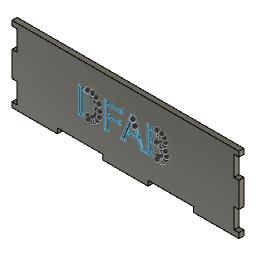
Component1 (Autodesk Fusion 360 design; units mm, degrees)
Autodesk Fusion 360 part; units mm, degrees
sketch "Sketch1" plane through (0, 0, 0) normal (0, 1, 0) x (1, 0, 0)
  line L0 (0, 0) -> (90, 0)
  line L1 (90, 0) -> (90, -30)
  line L2 (90, -30) -> (0, -30)
  line L3 (0, -30) -> (0, 0)
  line L4 (0, 0) -> (18, 0)
  line L5 (18, 0) -> (18, -2)
  line L6 (0, -2) -> (0, 0)
  line L7 (18, 0) -> (36, 0)
  line L8 (36, 0) -> (36, -2)
  line L9 (36, -2) -> (18, -2)
  line L10 (18, -2) -> (18, 0)
  line L11 (36, 0) -> (54, 0)
  line L12 (54, 0) -> (54, -2)
  line L13 (54, -2) -> (36, -2)
  line L14 (36, -2) -> (36, 0)
  line L15 (54, 0) -> (72, 0)
  line L16 (72, 0) -> (72, -2)
  line L17 (72, -2) -> (54, -2)
  line L18 (54, -2) -> (54, 0)
  line L19 (72, 0) -> (90, 0)
  line L20 (90, 0) -> (90, -2)
  line L21 (90, -2) -> (72, -2)
  line L22 (72, -2) -> (72, 0)
  line L23 (0, -30) -> (3, -30)
  line L24 (0, -30) -> (2, -30)
  line L25 (2, -30) -> (2, -20)
  line L26 (2, -20) -> (0, -20)
  line L27 (0, -20) -> (0, -30)
  line L28 (0, -20) -> (2, -20)
  line L29 (2, -20) -> (2, -10)
  line L30 (2, -10) -> (0, -10)
  line L31 (0, -10) -> (0, -20)
  line L32 (2, 0) -> (0, 0)
  line L33 (0, 0) -> (0, -10)
  line L34 (18, -2) -> (0, -2)
  line L35 (2, -10) -> (2, 0)
  line L36 (0, -10) -> (2, -10)
  line L37 (90, -30) -> (88, -30)
  line L38 (88, -30) -> (88, -20)
  line L39 (88, -20) -> (90, -20)
  line L40 (90, -20) -> (90, -30)
  line L41 (88, -20) -> (90, -20)
  line L42 (90, -20) -> (90, -10)
  line L43 (90, -10) -> (88, -10)
  line L44 (88, -10) -> (88, -20)
  line L45 (88, -10) -> (90, -10)
  line L46 (90, -10) -> (90, 0)
  line L47 (90, 0) -> (88, 0)
  line L48 (88, 0) -> (88, -10)
  line L49 (0, -30) -> (18, -30)
  line L50 (18, -30) -> (18, -28)
  line L51 (18, -28) -> (0, -28)
  line L52 (0, -28) -> (0, -30)
  line L53 (18, -30) -> (36, -30)
  line L54 (36, -30) -> (36, -28)
  line L55 (36, -28) -> (18, -28)
  line L56 (18, -28) -> (18, -30)
  line L57 (36, -30) -> (54, -30)
  line L58 (54, -30) -> (54, -28)
  line L59 (54, -28) -> (36, -28)
  line L60 (36, -28) -> (36, -30)
  line L61 (54, -30) -> (72, -30)
  line L62 (72, -30) -> (72, -28)
  line L63 (72, -28) -> (54, -28)
  line L64 (54, -28) -> (54, -30)
  line L65 (72, -30) -> (90, -30)
  line L66 (90, -30) -> (90, -28)
  line L67 (90, -28) -> (72, -28)
  line L68 (72, -28) -> (72, -30)
  dimension "d4" = 90
  dimension "d5" = 30
  dimension "d8" = 18
  dimension "d9" = 2
  dimension "d10" = 18
  dimension "d11" = 18
  dimension "d12" = 18
  dimension "d33" = 2
  dimension "d34" = 10
  dimension "d39" = 2
  dimension "d51" = 2
  dimension "d52" = 10
  dimension "d53" = 2
  dimension "d54" = 10
  dimension "d55" = 2
  dimension "d56" = 10
  dimension "d57" = 2
  dimension "d58" = 2
  dimension "d59" = 2
  dimension "d60" = 2
  dimension "d62" = 18
  dimension "d63" = 2
  dimension "d64" = 18
  dimension "d65" = 2
  dimension "d66" = 18
  dimension "d67" = 2
  dimension "d68" = 18
  dimension "d69" = 2
  dimension "d70" = 18
  dimension "d71" = 2
  constraint horizontal L0
  constraint vertical L1
  constraint horizontal L2
  constraint vertical L3
  constraint coincident L0.start L3.end
  constraint coincident L1 L20.end
  constraint horizontal L4
  constraint vertical L5
  constraint vertical L6
  constraint horizontal L7
  constraint vertical L8
  constraint horizontal L9
  constraint vertical L10
  constraint horizontal L11
  constraint vertical L12
  constraint horizontal L13
  constraint vertical L14
  constraint horizontal L15
  constraint vertical L16
  constraint horizontal L17
  constraint vertical L18
  constraint horizontal L19
  constraint vertical L20
  constraint horizontal L21
  constraint vertical L22
  constraint coincident L2 L23.end
  constraint coincident L0 L32.start
  constraint horizontal L24
  constraint vertical L25
  constraint horizontal L26
  constraint vertical L27
  constraint horizontal L28
  constraint vertical L29
  constraint horizontal L30
  constraint vertical L31
  constraint horizontal L32
  constraint vertical L33
  constraint perpendicular L6 L34
  constraint perpendicular L32 L35
  constraint horizontal L37
  constraint vertical L38
  constraint horizontal L39
  constraint vertical L40
  constraint horizontal L41
  constraint vertical L42
  constraint horizontal L43
  constraint vertical L44
  constraint horizontal L45
  constraint vertical L46
  constraint horizontal L47
  constraint vertical L48
  constraint horizontal L49
  constraint vertical L50
  constraint horizontal L51
  constraint vertical L52
  constraint horizontal L53
  constraint vertical L54
  constraint horizontal L55
  constraint vertical L56
  constraint horizontal L57
  constraint vertical L58
  constraint horizontal L59
  constraint vertical L60
  constraint horizontal L61
  constraint vertical L62
  constraint horizontal L63
  constraint vertical L64
  constraint horizontal L65
  constraint vertical L66
  constraint horizontal L67
  constraint vertical L68
  measures "d4" distance of L0.start L0.end
  measures "d5" distance of L0.start L2.end
  measures "d8" distance of L0.start L4.end
  measures "d9" distance of L0.start L6.start
  measures "d10" distance of L8 L10
  measures "d11" distance of L12 L14
  measures "d12" distance of L18 L22
  measures "d33" distance of L2.end L24.end
  measures "d34" distance of L2.end L26.end
  measures "d39" distance of L3 L29
  measures "d51" distance of L1.end L37.end
  measures "d52" distance of L1.end L39.end
  measures "d53" distance of L38.end L39.end
  measures "d54" distance of L38.end L43.end
  measures "d55" distance of L43.end L42.end
  measures "d56" distance of L43.end L47.end
  measures "d57" distance of L7 L9
  measures "d58" distance of L0 L13
  measures "d59" distance of L0 L17
  measures "d60" distance of L0 L21
  measures "d62" distance of L2.end L49.end
  measures "d63" distance of L2.end L51.end
  measures "d64" distance of L49.end L53.end
  measures "d65" distance of L49.end L50.end
  measures "d66" distance of L53.end L57.end
  measures "d67" distance of L53.end L54.end
  measures "d68" distance of L57.end L61.end
  measures "d69" distance of L57.end L58.end
  measures "d70" distance of L61.end L1.end
  measures "d71" distance of L61.end L62.end
extrude "Extrude2" add sketch "Sketch1" along normal blind 2 contours L0 L3 L4 L6 L32 L33 L34 L35 | L0 L4 L5 L10 L34 L35 | L9 L13 L17 L21 L25 L29 L34 L35 L38 L44 L48 L51 L55 L59 L63 L67 | L3 L26 L28 L29 L30 L31 L36 | L0 L8 L11 L12 L13 L14 L18 | L2 L3 L23 L24 L25 L27 L49 L51 L52 | L0 L16 L19 L21 L22 L48 | L2 L23 L25 L49 L50 L51 L56 | L0 L1 L19 L20 L21 L46 L47 L48 | L2 L50 L53 L54 L55 L56 L60 | L2 L54 L57 L58 L59 L60 L64 | L1 L39 L41 L42 L43 L44 L45 | L2 L58 L61 L62 L63 L64 L68 | L2 L38 L62 L65 L67 L68 | L1 L2 L37 L38 L40 L65 L66 L67
sketch "sketch 916" plane through (0, 0, 0) normal (0, -1, 0) x (1, 0, 0)
  line L0 (46.3643, 15.2561) -> (47.4625, 18.1893)
  spline S0 degree 2 poles (47.4625, 18.1893) (47.8104, 19.1375) (48.0014, 20.0993) knots -1 -1 -1 0 0 0
  spline S1 degree 2 poles (48.0014, 20.0993) (48.2333, 19.2875) (48.7108, 18.0256) knots -1 -1 -1 0 0 0
  line L1 (48.7108, 18.0256) -> (49.7545, 15.2561)
  line L2 (49.7545, 15.2561) -> (46.3643, 15.2561)
  line L3 (45.9823, 14.1784) -> (44.8841, 11.1497)
  line L4 (50.1637, 14.1784) -> (45.9823, 14.1784)
  line L5 (51.3302, 11.1497) -> (50.1637, 14.1784)
  line L6 (52.8377, 11.1497) -> (51.3302, 11.1497)
  line L7 (48.7449, 21.1497) -> (52.8377, 11.1497)
  line L8 (47.3193, 21.1497) -> (48.7449, 21.1497)
  line L9 (43.4789, 11.1497) -> (47.3193, 21.1497)
  line L10 (44.8841, 11.1497) -> (43.4789, 11.1497)
  line L11 (28.0491, 12.3298) -> (28.0491, 19.9697)
  line L12 (28.0491, 19.9697) -> (30.1501, 19.9697)
  spline S2 degree 2 poles (30.1501, 19.9697) (31.3302, 19.9697) (31.8622, 19.765) knots -1 -1 -1 0 0 0
  spline S3 degree 2 poles (31.8622, 19.765) (32.5989, 19.4785) (33.1139, 18.6361) knots -1 -1 -1 0 0 0
  spline S4 degree 2 poles (33.1139, 18.6361) (33.6289, 17.7937) (33.6289, 16.2248) knots -1 -1 -1 0 0 0
  spline S5 degree 2 poles (33.6289, 16.2248) (33.6289, 15.0924) (33.3663, 14.2978) knots -1 -1 -1 0 0 0
  spline S6 degree 2 poles (33.3663, 14.2978) (33.1037, 13.5031) (32.633, 13.0324) knots -1 -1 -1 0 0 0
  spline S7 degree 2 poles (32.633, 13.0324) (32.2988, 12.6982) (31.736, 12.514) knots -1 -1 -1 0 0 0
  spline S8 degree 2 poles (31.736, 12.514) (31.1733, 12.3298) (30.1842, 12.3298) knots -1 -1 -1 0 0 0
  line L13 (30.1842, 12.3298) -> (28.0491, 12.3298)
  spline S9 degree 2 poles (31.9407, 11.3203) (31.2415, 11.1497) (30.3343, 11.1497) knots 0 0 0 1 1 1
  spline S10 degree 2 poles (33.1344, 11.8216) (32.6399, 11.4908) (31.9407, 11.3203) knots 0 0 0 1 1 1
  spline S11 degree 2 poles (34.045, 12.7289) (33.6289, 12.1525) (33.1344, 11.8216) knots 0 0 0 1 1 1
  spline S12 degree 2 poles (34.7272, 14.1852) (34.4611, 13.3053) (34.045, 12.7289) knots 0 0 0 1 1 1
  spline S13 degree 2 poles (34.9932, 16.2043) (34.9932, 15.0652) (34.7272, 14.1852) knots 0 0 0 1 1 1
  spline S14 degree 2 poles (34.601, 18.5815) (34.9932, 17.5413) (34.9932, 16.2043) knots 0 0 0 1 1 1
  spline S15 degree 2 poles (33.4175, 20.2903) (34.2088, 19.6218) (34.601, 18.5815) knots 0 0 0 1 1 1
  spline S16 degree 2 poles (31.9509, 21.0065) (32.8104, 20.8087) (33.4175, 20.2903) knots 0 0 0 1 1 1
  spline S17 degree 2 poles (30.1706, 21.1497) (31.337, 21.1497) (31.9509, 21.0065) knots 0 0 0 1 1 1
  line L14 (26.7258, 21.1497) -> (30.1706, 21.1497)
  line L15 (26.7258, 11.1497) -> (26.7258, 21.1497)
  line L16 (30.3343, 11.1497) -> (26.7258, 11.1497)
  line L17 (38.206, 15.6927) -> (38.206, 11.1497)
  line L18 (42.8991, 15.6927) -> (38.206, 15.6927)
  line L19 (42.8991, 16.8728) -> (42.8991, 15.6927)
  line L20 (38.206, 16.8728) -> (42.8991, 16.8728)
  line L21 (38.206, 19.9697) -> (38.206, 16.8728)
  line L22 (43.6289, 19.9697) -> (38.206, 19.9697)
  line L23 (43.6289, 21.1497) -> (43.6289, 19.9697)
  line L24 (36.8827, 21.1497) -> (43.6289, 21.1497)
  line L25 (36.8827, 11.1497) -> (36.8827, 21.1497)
  line L26 (38.206, 11.1497) -> (36.8827, 11.1497)
  line L27 (55.1637, 16.9478) -> (55.1637, 19.9697)
  line L28 (55.1637, 19.9697) -> (57.1624, 19.9697)
  spline S18 degree 2 poles (57.1624, 19.9697) (58.2401, 19.9697) (58.6835, 19.8298) knots -1 -1 -1 0 0 0
  spline S19 degree 2 poles (58.6835, 19.8298) (59.1269, 19.69) (59.3656, 19.3114) knots -1 -1 -1 0 0 0
  spline S20 degree 2 poles (59.3656, 19.3114) (59.6044, 18.9328) (59.6044, 18.4349) knots -1 -1 -1 0 0 0
  spline S21 degree 2 poles (59.6044, 18.4349) (59.6044, 17.9096) (59.3486, 17.5617) knots -1 -1 -1 0 0 0
  spline S22 degree 2 poles (59.3486, 17.5617) (59.0928, 17.2139) (58.588, 17.0638) knots -1 -1 -1 0 0 0
  spline S23 degree 2 poles (58.588, 17.0638) (58.206, 16.9478) (57.3261, 16.9478) knots -1 -1 -1 0 0 0
  line L29 (57.3261, 16.9478) -> (55.1637, 16.9478)
  line L30 (55.1637, 12.3298) -> (55.1637, 15.7677)
  line L31 (55.1637, 15.7677) -> (57.4761, 15.7677)
  spline S24 degree 2 poles (57.4761, 15.7677) (58.4311, 15.7677) (58.9393, 15.6006) knots -1 -1 -1 0 0 0
  spline S25 degree 2 poles (58.9393, 15.6006) (59.4475, 15.4335) (59.734, 15.0208) knots -1 -1 -1 0 0 0
  spline S26 degree 2 poles (59.734, 15.0208) (60.0205, 14.6081) (60.0205, 14.0488) knots -1 -1 -1 0 0 0
  spline S27 degree 2 poles (60.0205, 14.0488) (60.0205, 13.5713) (59.8227, 13.2064) knots -1 -1 -1 0 0 0
  spline S28 degree 2 poles (59.8227, 13.2064) (59.6249, 12.8414) (59.3179, 12.6504) knots -1 -1 -1 0 0 0
  spline S29 degree 2 poles (59.3179, 12.6504) (59.0109, 12.4594) (58.5539, 12.3776) knots -1 -1 -1 0 0 0
  spline S30 degree 2 poles (58.5539, 12.3776) (58.2947, 12.3298) (57.6535, 12.3298) knots -1 -1 -1 0 0 0
  line L32 (57.6535, 12.3298) -> (55.1637, 12.3298)
  spline S31 degree 2 poles (59.2667, 11.3169) (58.6085, 11.1497) (57.6535, 11.1497) knots 0 0 0 1 1 1
  spline S32 degree 2 poles (60.3616, 11.8114) (59.925, 11.484) (59.2667, 11.3169) knots 0 0 0 1 1 1
  spline S33 degree 2 poles (61.0948, 12.7425) (60.7981, 12.1388) (60.3616, 11.8114) knots 0 0 0 1 1 1
  spline S34 degree 2 poles (61.3916, 14.0488) (61.3916, 13.3462) (61.0948, 12.7425) knots 0 0 0 1 1 1
  spline S35 degree 2 poles (60.9038, 15.5631) (61.3916, 14.9219) (61.3916, 14.0488) knots 0 0 0 1 1 1
  spline S36 degree 2 poles (59.5089, 16.4703) (60.4161, 16.2043) (60.9038, 15.5631) knots 0 0 0 1 1 1
  spline S37 degree 2 poles (60.5594, 17.3844) (60.2115, 16.8182) (59.5089, 16.4703) knots 0 0 0 1 1 1
  spline S38 degree 2 poles (60.9073, 18.5918) (60.9073, 17.9506) (60.5594, 17.3844) knots 0 0 0 1 1 1
  spline S39 degree 2 poles (60.515, 19.9117) (60.9073, 19.2807) (60.9073, 18.5918) knots 0 0 0 1 1 1
  spline S40 degree 2 poles (59.4304, 20.8462) (60.1228, 20.5426) (60.515, 19.9117) knots 0 0 0 1 1 1
  spline S41 degree 2 poles (57.5921, 21.1497) (58.7381, 21.1497) (59.4304, 20.8462) knots 0 0 0 1 1 1
  line L33 (53.8404, 21.1497) -> (57.5921, 21.1497)
  line L34 (53.8404, 11.1497) -> (53.8404, 21.1497)
  line L35 (57.6535, 11.1497) -> (53.8404, 11.1497)
extrude "Extrude3" cut sketch "sketch 916" against normal blind 1
equation "d4 = L"
equation "d5 = h"
equation "d8 = L / lt"
equation "d9 = e"
equation "d10 = d8"
equation "d11 = d10"
equation "d12 = d11"
equation "d17 = e"
equation "d33 = e"
equation "d34 = h / lh"
equation "d39 = d33"
equation "d51 = e"
equation "d52 = h / lh"
equation "d53 = e"
equation "d54 = h / lh"
equation "d55 = e"
equation "d56 = h / lh"
equation "d57 = e"
equation "d58 = e"
equation "d59 = e"
equation "d60 = e"
equation "d62 = d8"
equation "d63 = e"
equation "d64 = L / lt"
equation "d65 = e"
equation "d66 = d64"
equation "d67 = e"
equation "d68 = L / lt"
equation "d69 = e"
equation "d70 = L / lt"
equation "d71 = e"
equation "L = 90 mm"
equation "h = 30 mm"
equation "lt = 5"
equation "e = 2 mm"
equation "lh = 3"
